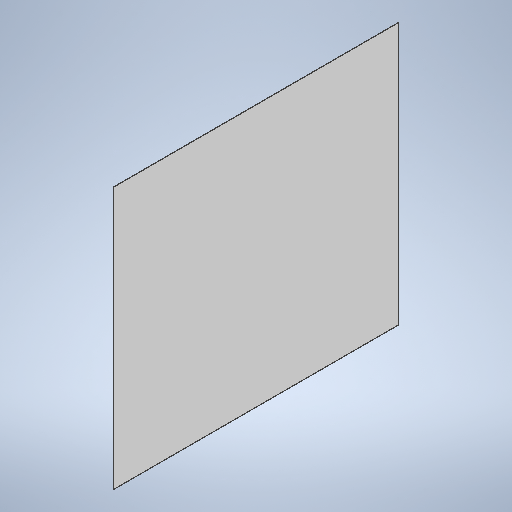
# Autodesk Inventor part: Деталь2
Saved by Autodesk Inventor 2026.2 (Build 302298000, 298)
## iProperties
Created: 2026-09-15
Part Number: Деталь2
Material: Generic
Document SubType Name: Sheet Metal
Designer: user
Density: 1 g/cm^3
Sheet Metal Rule: Default_mm
Appearance: Default
Mass: 3971.7 g
Surface Area: 39829.8 cm^2
Volume: 3971.7 cm^3
Flat Pattern Width: 135 cm
Flat Pattern Length: 147.1 cm
Flat Pattern Area: 19858.5 cm^2
Sheet Metal Width: 1350,000 mm
Sheet Metal Length: 1471,000 mm
Sheet Metal Area: 1985850,000 mm^2
Author: user
Autodesk Inventor part; units mm, degrees
ref_plane "YZ Plane" through (0, 0, 0) normal (1, 0, 0) x (0, 1, 0)
ref_plane "XZ Plane" through (0, 0, 0) normal (0, 1, 0) x (-1, 0, 0)
ref_plane "XY Plane" through (0, 0, 0) normal (0, 0, 1) x (1, 0, 0)
sketch "Эскиз1" plane through (0, 0, 0) normal (1, 0, 0) x (0, 1, 0)
  line L0 (-675, 735.5) -> (675, 735.5)
  line L1 (675, 735.5) -> (675, -735.5)
  line L2 (675, -735.5) -> (-675, -735.5)
  line L3 (-675, -735.5) -> (-675, 735.5)
  line L4 (-675, 735.5) -> (675, -735.5) construction
  line L5 (675, 735.5) -> (-675, -735.5) construction
  point P0 (0, 0)
  dimension "d0" = 1350
  dimension "d1" = 1471
  measures "d0" distance of L1.end L2.end
  measures "d1" distance of L0.end L1.end
extrude "Пластина1" add sketch "Эскиз1" along normal blind 2
equation "\"d2\" = Толщина"
equation "\"Радиус_гибки\" = Толщина"
equation "\"Ширина_просечки\" = Толщина"
equation "\"Глубина_просечки\" = 0.5 * Толщина"
equation "\"Размер_просечки\" = 4 * Толщина"
equation "\"Мин_остаток\" = 2 * Толщина"
equation "\"Радиус_перехода\" = Радиус_гибки"
equation "\"Радиус_Якоби\" = Радиус_гибки"
equation "\"Размер_зазора\" = Толщина"
equation "\"Толщина\" = 2"
